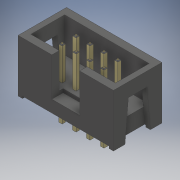
# Autodesk Inventor part: PinHeader_2x04_P2.54mm_Vertical_Shrouded
Saved by Autodesk Inventor 2017 (Build 210142000, 142)
## iProperties
Created: 2020-10-30
Part Number: PinHeader_2x04_P2.54mm_Vertical_Shrouded
Material: Generic
Document SubType Name: Modeling
Designer: Joe Ferner
Density: 1 g/cm^3
Appearance: Default
Author: Joe Ferner
Autodesk Inventor part; units mm, degrees
ref_plane "YZ Plane" through (0, 0, 0) normal (1, 0, 0) x (0, 1, 0)
ref_plane "XZ Plane" through (0, 0, 0) normal (0, 1, 0) x (-1, 0, 0)
sketch "Sketch1" plane through (0, 0, 0) normal (0, 1, 0) x (-1, 0, 0)
  line L0 (0, 0) -> (8.82, 0)
  line L1 (8.82, 0) -> (8.82, -17.37)
  line L2 (8.82, -17.37) -> (0, -17.37)
  line L3 (0, -17.37) -> (0, 0)
  dimension "length" = 17.37
  dimension "width" = 8.82
  constraints: 8 end point, 2 parallel, 1 horizontal, 1 perpendicular
  measures "length" distance of L2.end L0.start
  measures "width" distance of L0.start L0.end
extrude "Extrusion1" add sketch "Sketch1" along normal blind 9.57
sketch "Sketch2" plane through (0, 9.57, 0) normal (0, 1, 0) x (1, 0, 0)
  line L0 (-7.485, 0.99) -> (-1.335, 0.99)
  line L1 (-1.335, 0.99) -> (-1.335, 16.38)
  line L2 (-1.335, 16.38) -> (-7.485, 16.38)
  line L3 (-7.485, 16.38) -> (-7.485, 0.99)
  line L4 (0, 17.37) -> (-8.82, 17.37) projected
  line L5 (0, 0) -> (0, 17.37) projected
  dimension "d5" = 6.15
  dimension "d6" = 15.39
  dimension "d7" = 0.99
  dimension "d8" = 1.335
  constraints: 8 end point, 2 parallel, 1 horizontal, 1 perpendicular
  measures "d5" distance of L1.end L2.end
  measures "d6" distance of L0.end L1.end
  measures "d7" distance between parallel lines of L4 L2
  measures "d8" distance between parallel lines of L5 L1
extrude "Extrusion2" cut sketch "Sketch2" against normal blind 6.35
sketch "Sketch3" plane through (0, 9.57, 0) normal (0, 1, 0) x (1, 0, 0)
  line L0 (0, 0) -> (0, 17.37) projected
  line L1 (0, 6.145) -> (-2.0446, 6.145)
  line L2 (-2.0446, 6.145) -> (-2.0446, 11.225)
  line L3 (-2.0446, 11.225) -> (0, 11.225)
  line L4 (0, 11.225) -> (0, 6.145)
  line L5 (-8.82, 0) -> (0, 0) projected
  dimension "d11" = 5.08
  dimension "d12" = 6.145
  dimension "d13" = 2.0446
  constraints: 8 end point, 2 parallel, 1 horizontal, 1 perpendicular, 1 point on line
  measures "d11" distance between parallel lines of L3 L1
  measures "d12" distance between parallel lines of L5 L1
  measures "d13" distance of L1.start L1.end
extrude "Extrusion3" cut sketch "Sketch3" against normal blind 7
sketch "Sketch4" plane through (0, 0, 0) normal (0, -1, 0) x (1, 0, 0)
  line L0 (0, 0) -> (0, -17.37) projected
  line L1 (-8.82, -17.37) -> (-8.82, 0) projected
  line L2 (0, -0.8) -> (-8.82, -0.8)
  line L3 (-8.82, -0.8) -> (-8.82, -16.57)
  line L4 (-8.82, -16.57) -> (0, -16.57)
  line L5 (0, -16.57) -> (0, -0.8)
  line L6 (0, 0) -> (-8.82, 0) projected
  line L7 (-8.82, -17.37) -> (0, -17.37) projected
  dimension "d16" = 0.8
  dimension "d17" = 0.8
  constraints: 8 end point, 2 parallel, 2 point on line, 1 horizontal, 1 perpendicular
  measures "d16" distance between parallel lines of L6 L2
  measures "d17" distance between parallel lines of L7 L4
extrude "Extrusion4" cut sketch "Sketch4" against normal blind 0.38 contours L0 L4 L1 L2
sketch "Sketch5" plane through (-8.82, 0, 0) normal (0, 0, 1) x (1, 0, 0)
  line L0 (2.0915, 0) -> (2.71, 7.07)
  line L1 (2.71, 7.07) -> (6.11, 7.07)
  line L2 (6.11, 7.07) -> (6.7285, 0)
  line L3 (2.0915, 0) -> (6.7285, 0)
  line L4 (8.82, 0) -> (0, 0) projected
  line L5 (8.1271, 3.22) -> (11.7857, 3.22)
  line L6 (0, 9.57) -> (8.82, 9.57) projected
  dimension "width" = 8.82
  dimension "sideCutOutTopWidth" = 3.4
  dimension "d21" = 6.35
  dimension "d22" = 3.85
  dimension "d24" = 85
  dimension "d26" = 85
  dimension "d27" = 2.0915
  dimension "sideCutOutBottomWidth" = 4.6371
  constraints: 10 end point, 3 horizontal, 1 collinear
  measures "sideCutOutTopWidth" distance of L0.end L1.end
  measures "d21" distance between parallel lines of L6 L5
  measures "d22" distance between parallel lines of L1 L5
  measures "d24" angle of L3 L0
  measures "d26" angle of L3 L2
  measures "d27" distance of L4.end L0.start
  measures "sideCutOutBottomWidth" distance of L0.start L2.end
extrude "Extrusion5" cut sketch "Sketch5" against normal blind 1
ref_plane "Work Plane1" through (-8.82, 0, -8.685) normal (0, 0, 1) x (1, 0, 0)
mirror "Mirror1" about plane through (-8.82, 0, -8.685) normal (0, 0, 1) of "Extrusion5"
sketch "Sketch6" plane through (0, 3.22, 0) normal (0, 1, 0) x (1, 0, 0)
  line L0 (-2.83, 4.565) -> (-3.45, 4.565)
  line L1 (-3.45, 4.565) -> (-3.45, 5.185)
  line L2 (-3.45, 5.185) -> (-2.83, 5.185)
  line L3 (-2.83, 5.185) -> (-2.83, 4.565)
  line L4 (-2.83, 7.105) -> (-3.45, 7.105)
  line L5 (-3.45, 7.105) -> (-3.45, 7.725)
  line L6 (-3.45, 7.725) -> (-2.83, 7.725)
  line L7 (-2.83, 7.725) -> (-2.83, 7.105)
  line L8 (-2.83, 9.645) -> (-3.45, 9.645)
  line L9 (-3.45, 9.645) -> (-3.45, 10.265)
  line L10 (-3.45, 10.265) -> (-2.83, 10.265)
  line L11 (-2.83, 10.265) -> (-2.83, 9.645)
  line L12 (-2.83, 12.185) -> (-3.45, 12.185)
  line L13 (-3.45, 12.185) -> (-3.45, 12.805)
  line L14 (-3.45, 12.805) -> (-2.83, 12.805)
  line L15 (-2.83, 12.805) -> (-2.83, 12.185)
  line L16 (-5.37, 4.565) -> (-5.99, 4.565)
  line L17 (-5.99, 4.565) -> (-5.99, 5.185)
  line L18 (-5.99, 5.185) -> (-5.37, 5.185)
  line L19 (-5.37, 5.185) -> (-5.37, 4.565)
  line L20 (-5.37, 7.105) -> (-5.99, 7.105)
  line L21 (-5.99, 7.105) -> (-5.99, 7.725)
  line L22 (-5.99, 7.725) -> (-5.37, 7.725)
  line L23 (-5.37, 7.725) -> (-5.37, 7.105)
  line L24 (-5.37, 9.645) -> (-5.99, 9.645)
  line L25 (-5.99, 9.645) -> (-5.99, 10.265)
  line L26 (-5.99, 10.265) -> (-5.37, 10.265)
  line L27 (-5.37, 10.265) -> (-5.37, 9.645)
  line L28 (-5.37, 12.185) -> (-5.99, 12.185)
  line L29 (-5.99, 12.185) -> (-5.99, 12.805)
  line L30 (-5.99, 12.805) -> (-5.37, 12.805)
  line L31 (-5.37, 12.805) -> (-5.37, 12.185)
  line L32 (0, 0) -> (0, 6.145) projected
  line L33 (-8.82, 0) -> (0, 0) projected
  line L34 (-6.4732, 8.685) -> (-4.41, 8.685)
  line L35 (-4.41, 8.685) -> (-4.41, 4.7119)
  dimension "d31" = 0.62
  dimension "d32" = 0.62
  dimension "d35" = 2.54
  dimension "d38" = 2.54
  dimension "d43" = 0.96
  dimension "d44" = 0.96
  dimension "d45" = 4.41
  dimension "d46" = 8.685
  constraints: 68 end point, 3 horizontal, 2 collinear, 2 parallel, 2 perpendicular, 1 vertical, 54 other
  measures "d31" distance of L2.end L0.start
  measures "d32" distance of L0.start L0.end
  measures "d35" distance of L0.start L4.start
  measures "d38" distance of L0.start L16.start
  measures "d43" distance between parallel lines of L35 L23
  measures "d44" distance between parallel lines of L24 L34
  measures "d45" distance between parallel lines of L32 L35
  measures "d46" distance between parallel lines of L33 L34
extrude "Extrusion6" add sketch "Sketch6" along normal blind 6 and the other way blind 6.62
chamfer "Chamfer1" distance 0.15 angle 45 64 edges at (-5.68, 9.22, -4.565) (-5.37, 9.22, -4.875) (-5.68, 9.22, -5.185) (-5.99, 9.22, -4.875) (-3.45, 9.22, -4.875) (-3.14, 9.22, -5.185) (-2.83, 9.22, -4.875) (-3.14, 9.22, -4.565) (-3.14, 9.22, -7.105) (-2.83, 9.22, -7.415) (-3.14, 9.22, -7.725) (-3.45, 9.22, -7.415) (-5.37, 9.22, -7.415) (-5.68, 9.22, -7.105) (-5.99, 9.22, -7.415) (-5.68, 9.22, -7.725) (-5.68, 9.22, -9.645) (-5.37, 9.22, -9.955) (-5.68, 9.22, -10.265) (-5.99, 9.22, -9.955) (-5.68, 9.22, -12.185) (-5.37, 9.22, -12.495) (-5.68, 9.22, -12.805) (-5.99, 9.22, -12.495) (-2.83, 9.22, -9.955) (-3.14, 9.22, -9.645) (-3.45, 9.22, -9.955) (-3.14, 9.22, -10.265) (-3.14, 9.22, -12.185) (-2.83, 9.22, -12.495) (-3.14, 9.22, -12.805) (-3.45, 9.22, -12.495) (-2.83, -3.4, -4.875) (-3.14, -3.4, -5.185) (-3.45, -3.4, -4.875) (-3.14, -3.4, -4.565) (-5.37, -3.4, -4.875) (-5.68, -3.4, -4.565) (-5.99, -3.4, -4.875) (-5.68, -3.4, -5.185) (-5.68, -3.4, -7.105) (-5.37, -3.4, -7.415) (-5.99, -3.4, -7.415) (-5.68, -3.4, -7.725) (-3.45, -3.4, -7.415) (-2.83, -3.4, -7.415) (-3.14, -3.4, -7.105) (-3.14, -3.4, -7.725) (-2.83, -3.4, -9.955) (-3.14, -3.4, -9.645) (-3.45, -3.4, -9.955) (-3.14, -3.4, -10.265) (-5.37, -3.4, -9.955) (-5.68, -3.4, -9.645) (-5.99, -3.4, -9.955) (-5.68, -3.4, -10.265) (-5.68, -3.4, -12.185) (-5.99, -3.4, -12.495) (-5.37, -3.4, -12.495) (-5.68, -3.4, -12.805) (-3.45, -3.4, -12.495) (-3.14, -3.4, -12.185) (-3.14, -3.4, -12.805) (-2.83, -3.4, -12.495)
equation "\"d7\" = -0.5 * d6 + 0.5 * length"
equation "\"d8\" = -0.5 * d5 + 0.5 * width"
equation "\"d12\" = -0.5 * d11 + 0.5 * length"
equation "\"d27\" = -0.5 * sideCutOutBottomWidth + 0.5 * width"
equation "\"d45\" = 0.5 * width"
equation "\"d46\" = 0.5 * length"
body "Solid1"
